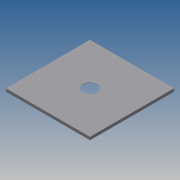
# Autodesk Inventor part: housingLid
Saved by Autodesk Inventor 2014 SP1 (Build 180222100, 222)
## iProperties
Created: 2014-03-12
Part Number: housingLid
Material: Generic
Document SubType Name: Modeling
Designer: Dave
Density: 1 g/cm^3
Appearance: Default
Author: Dave
Autodesk Inventor part; units mm, degrees
ref_plane "YZ Plane" through (0, 0, 0) normal (1, 0, 0) x (0, 1, 0)
ref_plane "XZ Plane" through (0, 0, 0) normal (0, 1, 0) x (-1, 0, 0)
ref_plane "XY Plane" through (0, 0, 0) normal (0, 0, 1) x (1, 0, 0)
sketch "Sketch1" plane through (0, 0, 0) normal (0, 1, 0) x (-1, 0, 0)
  line L0 (0, 0) -> (870, 0)
  line L1 (870, 0) -> (870, 870)
  line L2 (870, 870) -> (0, 870)
  line L3 (0, 870) -> (0, 0)
  dimension "d0" = 870
  dimension "d1" = 870
  constraints: 8 end point, 2 parallel, 1 horizontal, 1 perpendicular
  measures "d0" distance of L0.start L0.end
  measures "d1" distance of L2.end L0.start
extrude "Extrusion1" add sketch "Sketch1" along normal blind 30
sketch "Sketch2" plane through (0, 0, 0) normal (0, -1, 0) x (1, 0, 0)
  line L0 (0, 0) -> (-870, 0) projected
  line L1 (0, 870) -> (0, 0) projected
  line L2 (-870, 870) -> (0, 870) projected
  line L3 (-870, 0) -> (-870, 870) projected
  line L4 (-10, 860) -> (-10, 10)
  line L5 (-10, 10) -> (-860, 10)
  line L6 (-860, 10) -> (-860, 860)
  line L7 (-860, 860) -> (-10, 860)
  dimension "d4" = 10
  constraints: 8 end point, 3 other
  measures "d4" distance between parallel lines of L7 L2
extrude "Extrusion2" cut sketch "Sketch2" against normal blind 27.5 contours L4 L5 L6 L7
sketch "Sketch3" plane through (0, 30, 0) normal (0, 1, 0) x (1, 0, 0)
  circle A0 centre (-435, -435) radius 73.66
  line L0 (0, 0) -> (-870, 0) projected
  line L1 (-870, 0) -> (-870, -870) projected
  line L2 (-870, -870) -> (0, -870) projected
  line L3 (0, -870) -> (0, 0) projected
  line L4 (-435, 0) -> (-435, -870) construction
  line L5 (-870, -435) -> (0, -435) construction
  point P0 (-435, -435)
  dimension "d7" = 147.32
  constraints: 5 midpoint, 4 end point, 1 centre point, 1 coincident
  measures "d7" diameter of A0
extrude "Extrusion3" cut sketch "Sketch3" against normal blind 25.4 contours A0
body "Solid1"
